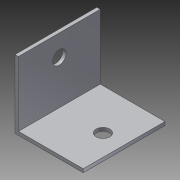
# Autodesk Inventor part: Hopper Pail Mounting Brace P13
Saved by Autodesk Inventor 2014 SP1 (Build 180222100, 222)
## iProperties
Created: 2013-12-17
Part Number: Hopper Pail Mounting Brace P13
Material: Aluminum 6061
Document SubType Name: Modeling
Designer: Moses
Mass: 1.23446 g
Surface Area: 12.4298 cm^2
Volume: 0.455519 cm^3
Density: 2.71 g/cm^3
Appearance: Aluminum - Flat
Author: Moses
Autodesk Inventor part; units mm, degrees
ref_plane "YZ Plane" through (0, 0, 0) normal (1, 0, 0) x (0, 1, 0)
ref_plane "XZ Plane" through (0, 0, 0) normal (0, 1, 0) x (-1, 0, 0)
sketch "Sketch1" plane through (0, 0, 0) normal (0, 0, 1) x (1, 0, 0)
  line L0 (0, 0) -> (0, 15.875)
  line L1 (0, 15.875) -> (0.7937, 15.875)
  line L2 (0.7937, 15.875) -> (0.7938, 0.7937)
  line L3 (0.7938, 0.7937) -> (15.875, 0.7937)
  line L4 (15.875, 0.7937) -> (15.875, 0)
  line L5 (15.875, 0) -> (0, 0)
  dimension "d0" = 15.875
  dimension "d1" = 0.7937
  dimension "d11" = 15.875
  constraints: 12 end point, 3 horizontal, 3 vertical, 1 perpendicular
  measures "d0" distance of L0.start L0.end
  measures "d1" distance of L0.end L1.end
  measures "d11" distance of L4.end L0.start
extrude "Extrusion1" add sketch "Sketch1" along normal blind 19.05
sketch "Sketch2" plane through (0.7938, 0.7937, 0) normal (1, 0, 0) x (0, 0, -1)
  line L0 (0, 15.0812) -> (0, 0) projected
  line L1 (-19.05, 0) -> (-19.05, 15.0812) projected
  circle A0 centre (-9.525, 10.16) radius 1.5875
  line L2 (0, 0) -> (-19.05, 0) projected
  line L3 (-19.05, 10.16) -> (0, 10.16) construction
  point P0 (0, -0.7937)
  dimension "d4" = 3.175
  dimension "d13" = 10.16
  constraints: 2 end point, 2 point on line, 1 centre point, 1 coincident, 1 horizontal, 1 midpoint
  measures "d4" diameter of A0
  measures "d13" distance from line of A0.centre L2
sketch "Sketch3" plane through (0.7938, 0.7937, 0) normal (0, 1, 0) x (1, 0, 0)
  line L0 (15.0812, -19.05) -> (0, -19.05) projected
  circle A0 centre (10.16, -9.525) radius 1.5875
  line L1 (0, 0) -> (0, -19.05) projected
  line L2 (10.16, 0) -> (10.16, -19.05) construction
  line L3 (0, 0) -> (15.0812, 0) projected
  point P0 (-0.7938, 0)
  dimension "d5" = 3.175
  dimension "d10" = 10.16
  dimension "d12" = 15.0813
  constraints: 2 end point, 2 point on line, 1 centre point, 1 coincident, 1 midpoint, 1 vertical
  measures "d5" diameter of A0
  measures "d10" distance between parallel lines of L2 L1
  measures "d12" distance of L1.start L3.end
extrude "Extrusion2" cut sketch "Sketch2" against normal through all
extrude "Extrusion3" cut sketch "Sketch3" against normal through all
ref_plane "Work Plane1" through (0, 0, 9.525) normal (0, 0, 1) x (1, 0, 0)
body "Solid1"
